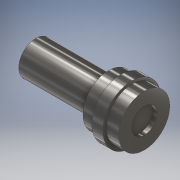
# Autodesk Inventor part: encoderaxis
Saved by Autodesk Inventor 2018.3 (Build 223284000, 284)
## iProperties
Created: 2019-09-29
Part Number: encoderaxis
Material: 一般
Document SubType Name: Modeling
Designer: Eiji Nishizawa
Density: 1 g/cm^3
Appearance: 鋼 - つや出し
Author: Eiji Nishizawa
Autodesk Inventor part; units mm, degrees
ref_plane "YZ Plane" through (0, 0, 0) normal (1, 0, 0) x (0, 1, 0)
ref_plane "XZ Plane" through (0, 0, 0) normal (0, 1, 0) x (-1, 0, 0)
ref_plane "XY Plane" through (0, 0, 0) normal (0, 0, 1) x (1, 0, 0)
sketch "スケッチ1" plane through (0, 0, 0) normal (1, 0, 0) x (0, 1, 0)
  circle A0 centre (0, 0) radius 4
  dimension "d0" = 8
  constraints: 1 centre point, 1 coincident
  measures "d0" diameter of A0
extrude "押し出し1" add sketch "スケッチ1" along normal blind 25.5
sketch "スケッチ2" plane through (25.5, 0, 0) normal (1, 0, 0) x (0, 0, -1)
  circle A0 centre (0, 0) radius 6
  circle A1 centre (0, 0) radius 4
  dimension "d3" = 12
  constraints: 2 centre point, 2 coincident
  measures "d3" diameter of A0
extrude "押し出し2" add sketch "スケッチ2" against normal blind 2.9
sketch "スケッチ3" plane through (22.6, 0, 0) normal (-1, 0, 0) x (0, 0, 1)
  circle A0 centre (0, 0) radius 3.6421
  circle A1 centre (-0.1483, 0) radius 6.8
  dimension "d6" = 13.6
  constraints: 2 centre point, 1 coincident
  measures "d6" diameter of A1
extrude "押し出し3" add sketch "スケッチ3" along normal blind 2.6
sketch "スケッチ4" plane through (20, 0, -0.1483) normal (-1, 0, 0) x (0, 0, 1)
  circle A0 centre (0.1483, 0) radius 4
  circle A1 centre (0.1483, 0) radius 6
  constraints: 2 centre point, 2 coincident
extrude "押し出し4" add sketch "スケッチ4" along normal blind 2.9
sketch "スケッチ5" plane through (25.5, 0, 0) normal (1, 0, 0) x (0, 0, -1)
  circle A0 centre (0, 0) radius 3
  dimension "d11" = 6
  constraints: 1 centre point, 1 coincident
  measures "d11" diameter of A0
extrude "押し出し5" cut sketch "スケッチ5" against normal blind 1
